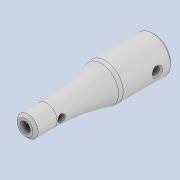
# Autodesk Inventor part: needle_conn_1
Saved by Autodesk Inventor 2020 (Build 240168000, 168)
## iProperties
Created: 2021-07-15
Part Number: needle_conn_1
Material: Generic
Document SubType Name: Modeling
Designer: Shuang Peng
Density: 1 g/cm^3
Appearance: Default
Author: Shuang Peng
Autodesk Inventor part; units mm, degrees
ref_plane "YZ Plane" through (0, 0, 0) normal (1, 0, 0) x (0, 1, 0)
ref_plane "XZ Plane" through (0, 0, 0) normal (0, 1, 0) x (-1, 0, 0)
ref_plane "XY Plane" through (0, 0, 0) normal (0, 0, 1) x (1, 0, 0)
sketch "Sketch1" plane through (0, 0, 0) normal (0, 0, 1) x (1, 0, 0)
  circle A0 centre (0, -6.4566) radius 1.5 projected
  circle A1 centre (0, -6.4566) radius 1.5
  circle A2 centre (0, -6.4566) radius 3.5
  point P0 (0, 0)
  dimension "d0" = 3
  dimension "d1" = 7
  constraints: 2 centre point, 2 coincident
  measures "d0" diameter of A1
  measures "d1" diameter of A2
extrude "Extrusion1" add sketch "Sketch1" along normal blind 8
sketch "Sketch2" plane through (0, -6.4566, 8) normal (0, 0, 1) x (1, 0, 0)
  circle A0 centre (0, 0) radius 3.5 projected
  point P0 (0, 6.4566)
extrude "Extrusion2" add sketch "Sketch2" along normal blind 2
sketch "Sketch3" plane through (0, -6.4566, 10) normal (0, 0, 1) x (1, 0, 0)
  circle A0 centre (0, 0) radius 3.5 projected
  circle A1 centre (0, 0) radius 1
  circle A2 centre (0, 0) radius 2
  point P0 (0, 6.4566)
  dimension "d6" = 2
  dimension "d7" = 4
  constraints: 2 centre point, 2 coincident
  measures "d6" diameter of A1
  measures "d7" diameter of A2
extrude "Extrusion3" add sketch "Sketch3" along normal blind 15 contours A2
fillet "Fillet1" radius 40 1 edges at (-2, -6.4566, 10)
fillet "Fillet2" radius 3 1 edges at (-3.5, -6.4566, 10)
chamfer "Chamfer1" distance 0.5 angle 45 1 edges at (-1.5, -6.4566, 0)
chamfer "Chamfer2" distance 0.5 angle 45 1 edges at (-2, -6.4566, 25)
sketch "Sketch4" plane through (0, 0, 0) normal (1, 0, 0) x (0, 1, 0)
  line L0 (-2.9566, 0) -> (-9.9566, 0) projected
  line L1 (-6.4566, 0) -> (-6.4566, 3)
  circle A0 centre (-6.4566, 3) radius 0.7
  point P0 (0, 0)
  dimension "d18" = 3
  dimension "d19" = 1.4
  constraints: 2 end point, 1 centre point, 1 coincident, 1 midpoint, 1 vertical
  measures "d18" distance of L1.start L1.end
  measures "d19" diameter of A0
extrude "Extrusion4" cut sketch "Sketch4" along normal mid plane 15
chamfer "Chamfer3" distance 0.3 angle 45 4 edges at (3.4625, -5.9454, 3.4781) (3.4627, -5.9468, 2.5204) (3.4293, -7.1566, 2.9993) (-3.4293, -7.1565, 2.9852)
chamfer "Chamfer4" distance 0.5 angle 45 1 edges at (-3.5, -6.4566, 0)
sketch "Sketch5" plane through (0, -6.4566, 10) normal (0, 0, 1) x (1, 0, 0)
  circle A0 centre (0, 0) radius 1 projected
  circle A1 centre (0, 0) radius 1
  point P0 (0, 6.4566)
  dimension "d28" = 2
  constraints: 1 centre point, 1 coincident
  measures "d28" diameter of A1
extrude "Extrusion5" cut sketch "Sketch5" against normal blind 10
sketch "Sketch6" plane through (0, 0, 0) normal (1, 0, 0) x (0, 1, 0)
  line L0 (-7.9566, 25) -> (-4.9566, 25) projected
  line L1 (-7.4566, 25) -> (-5.4566, 25) projected
  line L2 (-6.4566, 25) -> (-6.4566, 20)
  circle A0 centre (-6.4566, 20) radius 0.7
  point P0 (0, 0)
  dimension "d31" = 5
  dimension "d32" = 1.4
  constraints: 2 end point, 1 centre point, 1 coincident, 1 midpoint, 1 vertical
  measures "d31" distance of L2.start L2.end
  measures "d32" diameter of A0
extrude "Extrusion6" cut sketch "Sketch6" along normal mid plane 10
body "Solid1"
